Autodesk Inventor part; units mm, degrees
(part 9 of 15)
  arc A3906 (-13.7068, -39.825) -> (-13.6432, -39.825) centre (-13.675, -39.825) ccw
  arc A3907 (-13.6432, -38.375) -> (-13.7068, -38.375) centre (-13.675, -38.375) ccw
  arc A3908 (-15.8, -38.8) -> (-15.8, -38.6) centre (-15.8, -38.7) ccw
  arc A3909 (-15.8, -38.6) -> (-15.8, -38.8) centre (-15.8, -38.7) ccw
  line L1786 (-16.125, -36.575) -> (-13.675, -36.575)
  arc A3910 (-13.675, -36.6067) -> (-13.675, -36.5432) centre (-13.675, -36.575) ccw
  arc A3911 (-16.125, -36.5432) -> (-16.125, -36.6067) centre (-16.125, -36.575) ccw
  line L1787 (-13.675, -38.025) -> (-16.125, -38.025)
  arc A3912 (-16.125, -37.9932) -> (-16.125, -38.0567) centre (-16.125, -38.025) ccw
  arc A3913 (-13.675, -38.0567) -> (-13.675, -37.9932) centre (-13.675, -38.025) ccw
  line L1788 (-16.125, -38.025) -> (-16.125, -36.575)
  arc A3914 (-16.0933, -36.575) -> (-16.1568, -36.575) centre (-16.1251, -36.575) ccw
  arc A3915 (-16.1568, -38.025) -> (-16.0933, -38.025) centre (-16.1251, -38.025) ccw
  line L1789 (-13.675, -36.575) -> (-13.675, -38.025)
  arc A3916 (-13.7068, -38.025) -> (-13.6432, -38.025) centre (-13.675, -38.025) ccw
  arc A3917 (-13.6432, -36.575) -> (-13.7068, -36.575) centre (-13.675, -36.575) ccw
  arc A3918 (-15.8, -37) -> (-15.8, -36.8) centre (-15.8, -36.9) ccw
  arc A3919 (-15.8, -36.8) -> (-15.8, -37) centre (-15.8, -36.9) ccw
  line L1790 (-7.125, -38.375) -> (-4.675, -38.375)
  arc A3920 (-4.675, -38.4067) -> (-4.675, -38.3432) centre (-4.675, -38.375) ccw
  arc A3921 (-7.125, -38.3432) -> (-7.125, -38.4067) centre (-7.125, -38.375) ccw
  line L1791 (-4.675, -39.825) -> (-7.125, -39.825)
  arc A3922 (-7.125, -39.7932) -> (-7.125, -39.8567) centre (-7.125, -39.825) ccw
  arc A3923 (-4.675, -39.8567) -> (-4.675, -39.7932) centre (-4.675, -39.825) ccw
  line L1792 (-7.125, -39.825) -> (-7.125, -38.375)
  arc A3924 (-7.0933, -38.375) -> (-7.1568, -38.375) centre (-7.1251, -38.375) ccw
  arc A3925 (-7.1568, -39.825) -> (-7.0933, -39.825) centre (-7.1251, -39.825) ccw
  line L1793 (-4.675, -38.375) -> (-4.675, -39.825)
  arc A3926 (-4.7068, -39.825) -> (-4.6432, -39.825) centre (-4.675, -39.825) ccw
  arc A3927 (-4.6432, -38.375) -> (-4.7068, -38.375) centre (-4.675, -38.375) ccw
  arc A3928 (-6.8, -38.8) -> (-6.8, -38.6) centre (-6.8, -38.7) ccw
  arc A3929 (-6.8, -38.6) -> (-6.8, -38.8) centre (-6.8, -38.7) ccw
  line L1794 (-7.125, -36.575) -> (-4.675, -36.575)
  arc A3930 (-4.675, -36.6067) -> (-4.675, -36.5432) centre (-4.675, -36.575) ccw
  arc A3931 (-7.125, -36.5432) -> (-7.125, -36.6067) centre (-7.125, -36.575) ccw
  line L1795 (-4.675, -38.025) -> (-7.125, -38.025)
  arc A3932 (-7.125, -37.9932) -> (-7.125, -38.0567) centre (-7.125, -38.025) ccw
  arc A3933 (-4.675, -38.0567) -> (-4.675, -37.9932) centre (-4.675, -38.025) ccw
  line L1796 (-7.125, -38.025) -> (-7.125, -36.575)
  arc A3934 (-7.0933, -36.575) -> (-7.1568, -36.575) centre (-7.1251, -36.575) ccw
  arc A3935 (-7.1568, -38.025) -> (-7.0933, -38.025) centre (-7.1251, -38.025) ccw
  line L1797 (-4.675, -36.575) -> (-4.675, -38.025)
  arc A3936 (-4.7068, -38.025) -> (-4.6432, -38.025) centre (-4.675, -38.025) ccw
  arc A3937 (-4.6432, -36.575) -> (-4.7068, -36.575) centre (-4.675, -36.575) ccw
  arc A3938 (-6.8, -37) -> (-6.8, -36.8) centre (-6.8, -36.9) ccw
  arc A3939 (-6.8, -36.8) -> (-6.8, -37) centre (-6.8, -36.9) ccw
  line L1798 (15.725, -39.725) -> (13.275, -39.725)
  arc A3940 (13.275, -39.6932) -> (13.275, -39.7568) centre (13.275, -39.725) ccw
  arc A3941 (15.725, -39.7568) -> (15.725, -39.6932) centre (15.725, -39.725) ccw
  line L1799 (13.275, -38.275) -> (15.725, -38.275)
  arc A3942 (15.725, -38.3067) -> (15.725, -38.2432) centre (15.725, -38.275) ccw
  arc A3943 (13.275, -38.2432) -> (13.275, -38.3067) centre (13.275, -38.275) ccw
  line L1800 (15.725, -38.275) -> (15.725, -39.725)
  arc A3944 (15.6933, -39.725) -> (15.7568, -39.725) centre (15.725, -39.725) ccw
  arc A3945 (15.7568, -38.275) -> (15.6933, -38.275) centre (15.725, -38.275) ccw
  line L1801 (13.275, -39.725) -> (13.275, -38.275)
  arc A3946 (13.3068, -38.275) -> (13.2433, -38.275) centre (13.275, -38.275) ccw
  arc A3947 (13.2433, -39.725) -> (13.3068, -39.725) centre (13.275, -39.725) ccw
  arc A3948 (15.4, -39.5) -> (15.4, -39.3) centre (15.4, -39.4) ccw
  arc A3949 (15.4, -39.3) -> (15.4, -39.5) centre (15.4, -39.4) ccw
  line L1802 (15.725, -41.625) -> (13.275, -41.625)
  arc A3950 (13.275, -41.5932) -> (13.275, -41.6567) centre (13.275, -41.625) ccw
  arc A3951 (15.725, -41.6567) -> (15.725, -41.5932) centre (15.725, -41.625) ccw
  line L1803 (13.275, -40.175) -> (15.725, -40.175)
  arc A3952 (15.725, -40.2068) -> (15.725, -40.1433) centre (15.725, -40.1751) ccw
  arc A3953 (13.275, -40.1433) -> (13.275, -40.2068) centre (13.275, -40.1751) ccw
  line L1804 (15.725, -40.175) -> (15.725, -41.625)
  arc A3954 (15.6933, -41.625) -> (15.7568, -41.625) centre (15.725, -41.625) ccw
  arc A3955 (15.7568, -40.175) -> (15.6933, -40.175) centre (15.725, -40.175) ccw
  line L1805 (13.275, -41.625) -> (13.275, -40.175)
  arc A3956 (13.3068, -40.175) -> (13.2433, -40.175) centre (13.275, -40.175) ccw
  arc A3957 (13.2433, -41.625) -> (13.3068, -41.625) centre (13.275, -41.625) ccw
  arc A3958 (15.4, -41.4) -> (15.4, -41.2) centre (15.4, -41.3) ccw
  arc A3959 (15.4, -41.2) -> (15.4, -41.4) centre (15.4, -41.3) ccw
  line L1806 (-12.722, -87.325) -> (-12.722, -86.44)
  arc A3960 (-12.6839, -86.44) -> (-12.7601, -86.44) centre (-12.722, -86.44) ccw
  arc A3961 (-12.7601, -87.325) -> (-12.6839, -87.325) centre (-12.722, -87.325) ccw
  line L1807 (-9.878, -86.44) -> (-9.878, -87.325)
  arc A3962 (-9.9161, -87.325) -> (-9.8399, -87.325) centre (-9.878, -87.325) ccw
  arc A3963 (-9.8399, -86.44) -> (-9.9161, -86.44) centre (-9.878, -86.44) ccw
  line L1808 (-12.722, -86.44) -> (-12.018, -86.44)
  arc A3964 (-12.018, -86.4781) -> (-12.018, -86.4019) centre (-12.018, -86.44) ccw
  arc A3965 (-12.722, -86.4019) -> (-12.722, -86.4781) centre (-12.722, -86.44) ccw
  line L1809 (-10.948, -87.76) -> (-11.652, -87.76)
  arc A3966 (-11.652, -87.7219) -> (-11.652, -87.7981) centre (-11.652, -87.76) ccw
  arc A3967 (-10.948, -87.7981) -> (-10.948, -87.7219) centre (-10.948, -87.76) ccw
  line L1810 (-10.582, -86.44) -> (-9.878, -86.44)
  arc A3968 (-9.878, -86.4781) -> (-9.878, -86.4019) centre (-9.878, -86.44) ccw
  arc A3969 (-10.582, -86.4019) -> (-10.582, -86.4781) centre (-10.582, -86.44) ccw
  line L1811 (10.15, -94.475) -> (10.15, -95.125)
  arc A3970 (10.1119, -95.125) -> (10.1881, -95.125) centre (10.15, -95.125) ccw
  arc A3971 (10.1881, -94.475) -> (10.1119, -94.475) centre (10.15, -94.475) ccw
  line L1812 (8.45, -95.125) -> (8.45, -94.475)
  arc A3972 (8.4881, -94.475) -> (8.4119, -94.475) centre (8.45, -94.475) ccw
  arc A3973 (8.4119, -95.125) -> (8.4881, -95.125) centre (8.45, -95.125) ccw
  line L1813 (10.15, -95.125) -> (9.718, -95.125)
  arc A3974 (9.718, -95.0869) -> (9.718, -95.1631) centre (9.718, -95.125) ccw
  arc A3975 (10.15, -95.1631) -> (10.15, -95.0869) centre (10.15, -95.125) ccw
  line L1814 (9.248, -94.275) -> (9.352, -94.275)
  arc A3976 (9.352, -94.3131) -> (9.352, -94.2369) centre (9.352, -94.275) ccw
  arc A3977 (9.248, -94.2369) -> (9.248, -94.3131) centre (9.248, -94.275) ccw
  line L1815 (8.882, -95.125) -> (8.45, -95.125)
  arc A3978 (8.45, -95.0869) -> (8.45, -95.1631) centre (8.45, -95.125) ccw
  arc A3979 (8.882, -95.1631) -> (8.882, -95.0869) centre (8.882, -95.125) ccw
  line L1816 (-8.95, -105.475) -> (-8.95, -106.125)
  arc A3980 (-8.9881, -106.125) -> (-8.9119, -106.125) centre (-8.95, -106.125) ccw
  arc A3981 (-8.9119, -105.475) -> (-8.9881, -105.475) centre (-8.95, -105.475) ccw
  line L1817 (-10.65, -106.125) -> (-10.65, -105.475)
  arc A3982 (-10.6119, -105.475) -> (-10.6881, -105.475) centre (-10.65, -105.475) ccw
  arc A3983 (-10.6881, -106.125) -> (-10.6119, -106.125) centre (-10.65, -106.125) ccw
  line L1818 (-8.95, -106.125) -> (-9.382, -106.125)
  arc A3984 (-9.382, -106.0869) -> (-9.382, -106.1631) centre (-9.382, -106.125) ccw
  arc A3985 (-8.95, -106.1631) -> (-8.95, -106.0869) centre (-8.95, -106.125) ccw
  line L1819 (-9.852, -105.275) -> (-9.748, -105.275)
  arc A3986 (-9.748, -105.3131) -> (-9.748, -105.2369) centre (-9.748, -105.275) ccw
  arc A3987 (-9.852, -105.2369) -> (-9.852, -105.3131) centre (-9.852, -105.275) ccw
  line L1820 (-10.218, -106.125) -> (-10.65, -106.125)
  arc A3988 (-10.65, -106.0869) -> (-10.65, -106.1631) centre (-10.65, -106.125) ccw
  arc A3989 (-10.218, -106.1631) -> (-10.218, -106.0869) centre (-10.218, -106.125) ccw
  line L1821 (10.15, -92.575) -> (10.15, -93.225)
  arc A3990 (10.1119, -93.225) -> (10.1881, -93.225) centre (10.15, -93.225) ccw
  arc A3991 (10.1881, -92.575) -> (10.1119, -92.575) centre (10.15, -92.575) ccw
  line L1822 (8.45, -93.225) -> (8.45, -92.575)
  arc A3992 (8.4881, -92.575) -> (8.4119, -92.575) centre (8.45, -92.575) ccw
  arc A3993 (8.4119, -93.225) -> (8.4881, -93.225) centre (8.45, -93.225) ccw
  line L1823 (10.15, -93.225) -> (9.718, -93.225)
  arc A3994 (9.718, -93.1869) -> (9.718, -93.2631) centre (9.718, -93.225) ccw
  arc A3995 (10.15, -93.2631) -> (10.15, -93.1869) centre (10.15, -93.225) ccw
  line L1824 (9.248, -92.375) -> (9.352, -92.375)
  arc A3996 (9.352, -92.4131) -> (9.352, -92.3369) centre (9.352, -92.375) ccw
  arc A3997 (9.248, -92.3369) -> (9.248, -92.4131) centre (9.248, -92.375) ccw
  line L1825 (8.882, -93.225) -> (8.45, -93.225)
  arc A3998 (8.45, -93.1869) -> (8.45, -93.2631) centre (8.45, -93.225) ccw
  arc A3999 (8.882, -93.2631) -> (8.882, -93.1869) centre (8.882, -93.225) ccw
  line L1826 (-8.95, -107.475) -> (-8.95, -108.125)
  arc A4000 (-8.9881, -108.125) -> (-8.9119, -108.125) centre (-8.95, -108.125) ccw
  arc A4001 (-8.9119, -107.475) -> (-8.9881, -107.475) centre (-8.95, -107.475) ccw
  line L1827 (-10.65, -108.125) -> (-10.65, -107.475)
  arc A4002 (-10.6119, -107.475) -> (-10.6881, -107.475) centre (-10.65, -107.475) ccw
  arc A4003 (-10.6881, -108.125) -> (-10.6119, -108.125) centre (-10.65, -108.125) ccw
  line L1828 (-8.95, -108.125) -> (-9.382, -108.125)
  arc A4004 (-9.382, -108.0869) -> (-9.382, -108.1631) centre (-9.382, -108.125) ccw
  arc A4005 (-8.95, -108.1631) -> (-8.95, -108.0869) centre (-8.95, -108.125) ccw
  line L1829 (-9.852, -107.275) -> (-9.748, -107.275)
  arc A4006 (-9.748, -107.3131) -> (-9.748, -107.2369) centre (-9.748, -107.275) ccw
  arc A4007 (-9.852, -107.2369) -> (-9.852, -107.3131) centre (-9.852, -107.275) ccw
  line L1830 (-10.218, -108.125) -> (-10.65, -108.125)
  arc A4008 (-10.65, -108.0869) -> (-10.65, -108.1631) centre (-10.65, -108.125) ccw
  arc A4009 (-10.218, -108.1631) -> (-10.218, -108.0869) centre (-10.218, -108.125) ccw
  line L1831 (19.75, -91.825) -> (19.75, -91.175)
  arc A4010 (19.7881, -91.175) -> (19.7119, -91.175) centre (19.75, -91.175) ccw
  arc A4011 (19.7119, -91.825) -> (19.7881, -91.825) centre (19.75, -91.825) ccw
  line L1832 (21.45, -91.175) -> (21.45, -91.825)
  arc A4012 (21.4119, -91.825) -> (21.4881, -91.825) centre (21.45, -91.825) ccw
  arc A4013 (21.4881, -91.175) -> (21.4119, -91.175) centre (21.45, -91.175) ccw
  line L1833 (19.75, -91.175) -> (20.182, -91.175)
  arc A4014 (20.182, -91.2131) -> (20.182, -91.1369) centre (20.182, -91.175) ccw
  arc A4015 (19.75, -91.1369) -> (19.75, -91.2131) centre (19.75, -91.175) ccw
  line L1834 (20.652, -92.025) -> (20.548, -92.025)
  arc A4016 (20.548, -91.9869) -> (20.548, -92.0631) centre (20.548, -92.025) ccw
  arc A4017 (20.652, -92.0631) -> (20.652, -91.9869) centre (20.652, -92.025) ccw
  line L1835 (21.018, -91.175) -> (21.45, -91.175)
  arc A4018 (21.45, -91.2131) -> (21.45, -91.1369) centre (21.45, -91.175) ccw
  arc A4019 (21.018, -91.1369) -> (21.018, -91.2131) centre (21.018, -91.175) ccw
  line L1836 (19.75, -94.925) -> (19.75, -94.275)
  arc A4020 (19.7881, -94.275) -> (19.7119, -94.275) centre (19.75, -94.275) ccw
  arc A4021 (19.7119, -94.925) -> (19.7881, -94.925) centre (19.75, -94.925) ccw
  line L1837 (21.45, -94.275) -> (21.45, -94.925)
  arc A4022 (21.4119, -94.925) -> (21.4881, -94.925) centre (21.45, -94.925) ccw
  arc A4023 (21.4881, -94.275) -> (21.4119, -94.275) centre (21.45, -94.275) ccw
  line L1838 (19.75, -94.275) -> (20.182, -94.275)
  arc A4024 (20.182, -94.3131) -> (20.182, -94.2369) centre (20.182, -94.275) ccw
  arc A4025 (19.75, -94.2369) -> (19.75, -94.3131) centre (19.75, -94.275) ccw
  line L1839 (20.652, -95.125) -> (20.548, -95.125)
  arc A4026 (20.548, -95.0869) -> (20.548, -95.1631) centre (20.548, -95.125) ccw
  arc A4027 (20.652, -95.1631) -> (20.652, -95.0869) centre (20.652, -95.125) ccw
  line L1840 (21.018, -94.275) -> (21.45, -94.275)
  arc A4028 (21.45, -94.3131) -> (21.45, -94.2369) centre (21.45, -94.275) ccw
  arc A4029 (21.018, -94.2369) -> (21.018, -94.3131) centre (21.018, -94.275) ccw
  line L1841 (21.75, -94.925) -> (21.75, -94.275)
  arc A4030 (21.7881, -94.275) -> (21.7119, -94.275) centre (21.75, -94.275) ccw
  arc A4031 (21.7119, -94.925) -> (21.7881, -94.925) centre (21.75, -94.925) ccw
  line L1842 (23.45, -94.275) -> (23.45, -94.925)
  arc A4032 (23.4119, -94.925) -> (23.4881, -94.925) centre (23.45, -94.925) ccw
  arc A4033 (23.4881, -94.275) -> (23.4119, -94.275) centre (23.45, -94.275) ccw
  line L1843 (21.75, -94.275) -> (22.182, -94.275)
  arc A4034 (22.182, -94.3131) -> (22.182, -94.2369) centre (22.182, -94.275) ccw
  arc A4035 (21.75, -94.2369) -> (21.75, -94.3131) centre (21.75, -94.275) ccw
  line L1844 (22.652, -95.125) -> (22.548, -95.125)
  arc A4036 (22.548, -95.0869) -> (22.548, -95.1631) centre (22.548, -95.125) ccw
  arc A4037 (22.652, -95.1631) -> (22.652, -95.0869) centre (22.652, -95.125) ccw
  line L1845 (23.018, -94.275) -> (23.45, -94.275)
  arc A4038 (23.45, -94.3131) -> (23.45, -94.2369) centre (23.45, -94.275) ccw
  arc A4039 (23.018, -94.2369) -> (23.018, -94.3131) centre (23.018, -94.275) ccw
  line L1846 (21.75, -91.825) -> (21.75, -91.175)
  arc A4040 (21.7881, -91.175) -> (21.7119, -91.175) centre (21.75, -91.175) ccw
  arc A4041 (21.7119, -91.825) -> (21.7881, -91.825) centre (21.75, -91.825) ccw
  line L1847 (23.45, -91.175) -> (23.45, -91.825)
  arc A4042 (23.4119, -91.825) -> (23.4881, -91.825) centre (23.45, -91.825) ccw
  arc A4043 (23.4881, -91.175) -> (23.4119, -91.175) centre (23.45, -91.175) ccw
  line L1848 (21.75, -91.175) -> (22.182, -91.175)
  arc A4044 (22.182, -91.2131) -> (22.182, -91.1369) centre (22.182, -91.175) ccw
  arc A4045 (21.75, -91.1369) -> (21.75, -91.2131) centre (21.75, -91.175) ccw
  line L1849 (22.652, -92.025) -> (22.548, -92.025)
  arc A4046 (22.548, -91.9869) -> (22.548, -92.0631) centre (22.548, -92.025) ccw
  arc A4047 (22.652, -92.0631) -> (22.652, -91.9869) centre (22.652, -92.025) ccw
  line L1850 (23.018, -91.175) -> (23.45, -91.175)
  arc A4048 (23.45, -91.2131) -> (23.45, -91.1369) centre (23.45, -91.175) ccw
  arc A4049 (23.018, -91.1369) -> (23.018, -91.2131) centre (23.018, -91.175) ccw
  line L1851 (-55.4108, -61.543) -> (-60.3892, -61.543)
  arc A4050 (-60.3892, -61.4922) -> (-60.3892, -61.5938) centre (-60.3892, -61.543) ccw
  arc A4051 (-55.4108, -61.5938) -> (-55.4108, -61.4922) centre (-55.4108, -61.543) ccw
  line L1852 (-60.3892, -61.543) -> (-60.3892, -59.257)
  arc A4052 (-60.3384, -59.257) -> (-60.44, -59.257) centre (-60.3892, -59.257) ccw
  arc A4053 (-60.44, -61.543) -> (-60.3384, -61.543) centre (-60.3892, -61.543) ccw
  line L1853 (-60.3892, -59.257) -> (-55.4108, -59.257)
  arc A4054 (-55.4108, -59.3078) -> (-55.4108, -59.2062) centre (-55.4108, -59.257) ccw
  arc A4055 (-60.3892, -59.2062) -> (-60.3892, -59.3078) centre (-60.3892, -59.257) ccw
  line L1854 (-55.4108, -59.257) -> (-55.4108, -61.543)
  arc A4056 (-55.4616, -61.543) -> (-55.36, -61.543) centre (-55.4108, -61.543) ccw
  arc A4057 (-55.36, -59.257) -> (-55.4616, -59.257) centre (-55.4108, -59.257) ccw
  line L1855 (-10.2542, 51.989) -> (-6.5458, 51.989)
  arc A4058 (-6.5458, 51.9382) -> (-6.5458, 52.0398) centre (-6.5458, 51.989) ccw
  arc A4059 (-10.2542, 52.0398) -> (-10.2542, 51.9382) centre (-10.2542, 51.989) ccw
  line L1856 (-6.5458, 51.989) -> (-6.5458, 50.211)
  arc A4060 (-6.5966, 50.211) -> (-6.495, 50.211) centre (-6.5458, 50.211) ccw
  arc A4061 (-6.495, 51.989) -> (-6.5966, 51.989) centre (-6.5458, 51.989) ccw
  line L1857 (-6.5458, 50.211) -> (-10.2542, 50.211)
  arc A4062 (-10.2542, 50.2618) -> (-10.2542, 50.1602) centre (-10.2542, 50.211) ccw
  arc A4063 (-6.5458, 50.1602) -> (-6.5458, 50.2618) centre (-6.5458, 50.211) ccw
  line L1858 (-10.2542, 50.211) -> (-10.2542, 51.989)
  arc A4064 (-10.2034, 51.989) -> (-10.305, 51.989) centre (-10.2542, 51.989) ccw
  arc A4065 (-10.305, 50.211) -> (-10.2034, 50.211) centre (-10.2542, 50.211) ccw
  line L1859 (-7.692, -83.684) -> (-7.692, -85.716)
  arc A4066 (-7.7428, -85.716) -> (-7.6412, -85.716) centre (-7.692, -85.716) ccw
  arc A4067 (-7.6412, -83.684) -> (-7.7428, -83.684) centre (-7.692, -83.684) ccw
  line L1860 (-7.692, -85.716) -> (-8.708, -85.716)
  arc A4068 (-8.708, -85.6652) -> (-8.708, -85.7668) centre (-8.708, -85.716) ccw
  arc A4069 (-7.692, -85.7668) -> (-7.692, -85.6652) centre (-7.692, -85.716) ccw
  line L1861 (-8.708, -85.716) -> (-8.708, -83.684)
  arc A4070 (-8.6572, -83.684) -> (-8.7588, -83.684) centre (-8.708, -83.684) ccw
  arc A4071 (-8.7588, -85.716) -> (-8.6572, -85.716) centre (-8.708, -85.716) ccw
  line L1862 (-8.708, -83.684) -> (-7.692, -83.684)
  arc A4072 (-7.692, -83.7348) -> (-7.692, -83.6332) centre (-7.692, -83.684) ccw
  arc A4073 (-8.708, -83.6332) -> (-8.708, -83.7348) centre (-8.708, -83.684) ccw
  line L1863 (-5.5458, -87.889) -> (-9.2542, -87.889)
  arc A4074 (-9.2542, -87.8382) -> (-9.2542, -87.9398) centre (-9.2542, -87.889) ccw
  arc A4075 (-5.5458, -87.9398) -> (-5.5458, -87.8382) centre (-5.5458, -87.889) ccw
  line L1864 (-9.2542, -87.889) -> (-9.2542, -86.111)
  arc A4076 (-9.2034, -86.111) -> (-9.305, -86.111) centre (-9.2542, -86.111) ccw
  arc A4077 (-9.305, -87.889) -> (-9.2034, -87.889) centre (-9.2542, -87.889) ccw
  line L1865 (-9.2542, -86.111) -> (-5.5458, -86.111)
  arc A4078 (-5.5458, -86.1618) -> (-5.5458, -86.0602) centre (-5.5458, -86.111) ccw
  arc A4079 (-9.2542, -86.0602) -> (-9.2542, -86.1618) centre (-9.2542, -86.111) ccw
  line L1866 (-5.5458, -86.111) -> (-5.5458, -87.889)
  arc A4080 (-5.5966, -87.889) -> (-5.495, -87.889) centre (-5.5458, -87.889) ccw
  arc A4081 (-5.495, -86.111) -> (-5.5966, -86.111) centre (-5.5458, -86.111) ccw
  line L1867 (-13.392, -87.984) -> (-13.392, -90.016)
  arc A4082 (-13.4428, -90.016) -> (-13.3412, -90.016) centre (-13.392, -90.016) ccw
  arc A4083 (-13.3412, -87.984) -> (-13.4428, -87.984) centre (-13.392, -87.984) ccw
  line L1868 (-13.392, -90.016) -> (-14.408, -90.016)
  arc A4084 (-14.408, -89.9652) -> (-14.408, -90.0668) centre (-14.408, -90.016) ccw
  arc A4085 (-13.392, -90.0668) -> (-13.392, -89.9652) centre (-13.392, -90.016) ccw
  line L1869 (-14.408, -90.016) -> (-14.408, -87.984)
  arc A4086 (-14.3572, -87.984) -> (-14.4588, -87.984) centre (-14.408, -87.984) ccw
  arc A4087 (-14.4588, -90.016) -> (-14.3572, -90.016) centre (-14.408, -90.016) ccw
  line L1870 (-14.408, -87.984) -> (-13.392, -87.984)
  arc A4088 (-13.392, -88.0348) -> (-13.392, -87.9332) centre (-13.392, -87.984) ccw
  arc A4089 (-14.408, -87.9332) -> (-14.408, -88.0348) centre (-14.408, -87.984) ccw
  line L1871 (-9.3458, -90.889) -> (-13.0542, -90.889)
  arc A4090 (-13.0542, -90.8382) -> (-13.0542, -90.9398) centre (-13.0542, -90.889) ccw
  arc A4091 (-9.3458, -90.9398) -> (-9.3458, -90.8382) centre (-9.3458, -90.889) ccw
  line L1872 (-13.0542, -90.889) -> (-13.0542, -89.111)
  arc A4092 (-13.0034, -89.111) -> (-13.105, -89.111) centre (-13.0542, -89.111) ccw
  arc A4093 (-13.105, -90.889) -> (-13.0034, -90.889) centre (-13.0542, -90.889) ccw
  line L1873 (-13.0542, -89.111) -> (-9.3458, -89.111)
  arc A4094 (-9.3458, -89.1618) -> (-9.3458, -89.0602) centre (-9.3458, -89.111) ccw
  arc A4095 (-13.0542, -89.0602) -> (-13.0542, -89.1618) centre (-13.0542, -89.111) ccw
  line L1874 (-9.3458, -89.111) -> (-9.3458, -90.889)
  arc A4096 (-9.3966, -90.889) -> (-9.295, -90.889) centre (-9.3458, -90.889) ccw
  arc A4097 (-9.295, -89.111) -> (-9.3966, -89.111) centre (-9.3458, -89.111) ccw
  line L1875 (-13.303, -97.035) -> (-16.097, -97.035)
  arc A4098 (-16.097, -96.9842) -> (-16.097, -97.0858) centre (-16.097, -97.035) ccw
  arc A4099 (-13.303, -97.0858) -> (-13.303, -96.9842) centre (-13.303, -97.035) ccw
  line L1876 (-16.097, -97.035) -> (-16.097, -95.765)
  arc A4100 (-16.0462, -95.765) -> (-16.1478, -95.765) centre (-16.097, -95.765) ccw
  arc A4101 (-16.1478, -97.035) -> (-16.0462, -97.035) centre (-16.097, -97.035) ccw
  line L1877 (-16.097, -95.765) -> (-13.303, -95.765)
  arc A4102 (-13.303, -95.8158) -> (-13.303, -95.7142) centre (-13.303, -95.765) ccw
  arc A4103 (-16.097, -95.7142) -> (-16.097, -95.8158) centre (-16.097, -95.765) ccw
  line L1878 (-13.303, -95.765) -> (-13.303, -97.035)
  arc A4104 (-13.3538, -97.035) -> (-13.2522, -97.035) centre (-13.303, -97.035) ccw
  arc A4105 (-13.2522, -95.765) -> (-13.3538, -95.765) centre (-13.303, -95.765) ccw
  line L1879 (-18.316, -98.092) -> (-16.284, -98.092)
  arc A4106 (-16.284, -98.1428) -> (-16.284, -98.0412) centre (-16.284, -98.092) ccw
  arc A4107 (-18.316, -98.0412) -> (-18.316, -98.1428) centre (-18.316, -98.092) ccw
  line L1880 (-16.284, -98.092) -> (-16.284, -99.108)
  arc A4108 (-16.3348, -99.108) -> (-16.2332, -99.108) centre (-16.284, -99.108) ccw
  arc A4109 (-16.2332, -98.092) -> (-16.3348, -98.092) centre (-16.284, -98.092) ccw
  line L1881 (-16.284, -99.108) -> (-18.316, -99.108)
  arc A4110 (-18.316, -99.0572) -> (-18.316, -99.1588) centre (-18.316, -99.108) ccw
  arc A4111 (-16.284, -99.1588) -> (-16.284, -99.0572) centre (-16.284, -99.108) ccw
  line L1882 (-18.316, -99.108) -> (-18.316, -98.092)
  arc A4112 (-18.2652, -98.092) -> (-18.3668, -98.092) centre (-18.316, -98.092) ccw
  arc A4113 (-18.3668, -99.108) -> (-18.2652, -99.108) centre (-18.316, -99.108) ccw
  line L1883 (-17.284, -103.108) -> (-19.316, -103.108)
  arc A4114 (-19.316, -103.0572) -> (-19.316, -103.1588) centre (-19.316, -103.108) ccw
  arc A4115 (-17.284, -103.1588) -> (-17.284, -103.0572) centre (-17.284, -103.108) ccw
  line L1884 (-19.316, -103.108) -> (-19.316, -102.092)
  arc A4116 (-19.2652, -102.092) -> (-19.3668, -102.092) centre (-19.316, -102.092) ccw
  arc A4117 (-19.3668, -103.108) -> (-19.2652, -103.108) centre (-19.316, -103.108) ccw
  line L1885 (-19.316, -102.092) -> (-17.284, -102.092)
  arc A4118 (-17.284, -102.1428) -> (-17.284, -102.0412) centre (-17.284, -102.092) ccw
  arc A4119 (-19.316, -102.0412) -> (-19.316, -102.1428) centre (-19.316, -102.092) ccw
  line L1886 (-17.284, -102.092) -> (-17.284, -103.108)
  arc A4120 (-17.3348, -103.108) -> (-17.2332, -103.108) centre (-17.284, -103.108) ccw
  arc A4121 (-17.2332, -102.092) -> (-17.3348, -102.092) centre (-17.284, -102.092) ccw
  line L1887 (-17.308, -105.116) -> (-17.308, -103.084)
  arc A4122 (-17.2572, -103.084) -> (-17.3588, -103.084) centre (-17.308, -103.084) ccw
  arc A4123 (-17.3588, -105.116) -> (-17.2572, -105.116) centre (-17.308, -105.116) ccw
  line L1888 (-17.308, -103.084) -> (-16.292, -103.084)
  arc A4124 (-16.292, -103.1348) -> (-16.292, -103.0332) centre (-16.292, -103.084) ccw
  arc A4125 (-17.308, -103.0332) -> (-17.308, -103.1348) centre (-17.308, -103.084) ccw
  line L1889 (-16.292, -103.084) -> (-16.292, -105.116)
  arc A4126 (-16.3428, -105.116) -> (-16.2412, -105.116) centre (-16.292, -105.116) ccw
  arc A4127 (-16.2412, -103.084) -> (-16.3428, -103.084) centre (-16.292, -103.084) ccw
  line L1890 (-16.292, -105.116) -> (-17.308, -105.116)
  arc A4128 (-17.308, -105.0652) -> (-17.308, -105.1668) centre (-17.308, -105.116) ccw
  arc A4129 (-16.292, -105.1668) -> (-16.292, -105.0652) centre (-16.292, -105.116) ccw
  line L1891 (-19.308, -105.116) -> (-19.308, -103.084)
  arc A4130 (-19.2572, -103.084) -> (-19.3588, -103.084) centre (-19.308, -103.084) ccw
  arc A4131 (-19.3588, -105.116) -> (-19.2572, -105.116) centre (-19.308, -105.116) ccw
  line L1892 (-19.308, -103.084) -> (-18.292, -103.084)
  arc A4132 (-18.292, -103.1348) -> (-18.292, -103.0332) centre (-18.292, -103.084) ccw
  arc A4133 (-19.308, -103.0332) -> (-19.308, -103.1348) centre (-19.308, -103.084) ccw
  line L1893 (-18.292, -103.084) -> (-18.292, -105.116)
  arc A4134 (-18.3428, -105.116) -> (-18.2412, -105.116) centre (-18.292, -105.116) ccw
  arc A4135 (-18.2412, -103.084) -> (-18.3428, -103.084) centre (-18.292, -103.084) ccw
  line L1894 (-18.292, -105.116) -> (-19.308, -105.116)
  arc A4136 (-19.308, -105.0652) -> (-19.308, -105.1668) centre (-19.308, -105.116) ccw
  arc A4137 (-18.292, -105.1668) -> (-18.292, -105.0652) centre (-18.292, -105.116) ccw
  line L1895 (-19.308, -102.116) -> (-19.308, -100.084)
  arc A4138 (-19.2572, -100.084) -> (-19.3588, -100.084) centre (-19.308, -100.084) ccw
  arc A4139 (-19.3588, -102.116) -> (-19.2572, -102.116) centre (-19.308, -102.116) ccw
  line L1896 (-19.308, -100.084) -> (-18.292, -100.084)
  arc A4140 (-18.292, -100.1348) -> (-18.292, -100.0332) centre (-18.292, -100.084) ccw
  arc A4141 (-19.308, -100.0332) -> (-19.308, -100.1348) centre (-19.308, -100.084) ccw
  line L1897 (-18.292, -100.084) -> (-18.292, -102.116)
  arc A4142 (-18.3428, -102.116) -> (-18.2412, -102.116) centre (-18.292, -102.116) ccw
  arc A4143 (-18.2412, -100.084) -> (-18.3428, -100.084) centre (-18.292, -100.084) ccw
  line L1898 (-18.292, -102.116) -> (-19.308, -102.116)
  arc A4144 (-19.308, -102.0652) -> (-19.308, -102.1668) centre (-19.308, -102.116) ccw
  arc A4145 (-18.292, -102.1668) -> (-18.292, -102.0652) centre (-18.292, -102.116) ccw
  line L1899 (-18.308, -98.116) -> (-18.308, -96.084)
  arc A4146 (-18.2572, -96.084) -> (-18.3588, -96.084) centre (-18.308, -96.084) ccw
  arc A4147 (-18.3588, -98.116) -> (-18.2572, -98.116) centre (-18.308, -98.116) ccw
  line L1900 (-18.308, -96.084) -> (-17.292, -96.084)
  arc A4148 (-17.292, -96.1348) -> (-17.292, -96.0332) centre (-17.292, -96.084) ccw
  arc A4149 (-18.308, -96.0332) -> (-18.308, -96.1348) centre (-18.308, -96.084) ccw
  line L1901 (-17.292, -96.084) -> (-17.292, -98.116)
  arc A4150 (-17.3428, -98.116) -> (-17.2412, -98.116) centre (-17.292, -98.116) ccw
  arc A4151 (-17.2412, -96.084) -> (-17.3428, -96.084) centre (-17.292, -96.084) ccw
  line L1902 (-17.292, -98.116) -> (-18.308, -98.116)
  arc A4152 (-18.308, -98.0652) -> (-18.308, -98.1668) centre (-18.308, -98.116) ccw
  arc A4153 (-17.292, -98.1668) -> (-17.292, -98.0652) centre (-17.292, -98.116) ccw
  line L1903 (-16.208, -105.116) -> (-16.208, -103.084)
  arc A4154 (-16.1572, -103.084) -> (-16.2588, -103.084) centre (-16.208, -103.084) ccw
  arc A4155 (-16.2588, -105.116) -> (-16.1572, -105.116) centre (-16.208, -105.116) ccw
  line L1904 (-16.208, -103.084) -> (-15.192, -103.084)
  arc A4156 (-15.192, -103.1348) -> (-15.192, -103.0332) centre (-15.192, -103.084) ccw
  arc A4157 (-16.208, -103.0332) -> (-16.208, -103.1348) centre (-16.208, -103.084) ccw
  line L1905 (-15.192, -103.084) -> (-15.192, -105.116)
  arc A4158 (-15.2428, -105.116) -> (-15.1412, -105.116) centre (-15.192, -105.116) ccw
  arc A4159 (-15.1412, -103.084) -> (-15.2428, -103.084) centre (-15.192, -103.084) ccw
  line L1906 (-15.192, -105.116) -> (-16.208, -105.116)
  arc A4160 (-16.208, -105.0652) -> (-16.208, -105.1668) centre (-16.208, -105.116) ccw
  arc A4161 (-15.192, -105.1668) -> (-15.192, -105.0652) centre (-15.192, -105.116) ccw
  line L1907 (-8.365, -97.203) -> (-8.365, -99.997)
  arc A4162 (-8.4158, -99.997) -> (-8.3142, -99.997) centre (-8.365, -99.997) ccw
  arc A4163 (-8.3142, -97.203) -> (-8.4158, -97.203) centre (-8.365, -97.203) ccw
  line L1908 (-8.365, -99.997) -> (-9.635, -99.997)
  arc A4164 (-9.635, -99.9462) -> (-9.635, -100.0478) centre (-9.635, -99.997) ccw
  arc A4165 (-8.365, -100.0478) -> (-8.365, -99.9462) centre (-8.365, -99.997) ccw
  line L1909 (-9.635, -99.997) -> (-9.635, -97.203)
  arc A4166 (-9.5842, -97.203) -> (-9.6858, -97.203) centre (-9.635, -97.203) ccw
  arc A4167 (-9.6858, -99.997) -> (-9.5842, -99.997) centre (-9.635, -99.997) ccw
  line L1910 (-9.635, -97.203) -> (-8.365, -97.203)
  arc A4168 (-8.365, -97.2538) -> (-8.365, -97.1522) centre (-8.365, -97.203) ccw
  arc A4169 (-9.635, -97.1522) -> (-9.635, -97.2538) centre (-9.635, -97.203) ccw
  line L1911 (-10.2542, 50.189) -> (-6.5458, 50.189)
  arc A4170 (-6.5458, 50.1382) -> (-6.5458, 50.2398) centre (-6.5458, 50.189) ccw
  arc A4171 (-10.2542, 50.2398) -> (-10.2542, 50.1382) centre (-10.2542, 50.189) ccw
  line L1912 (-6.5458, 50.189) -> (-6.5458, 48.411)
  arc A4172 (-6.5966, 48.411) -> (-6.495, 48.411) centre (-6.5458, 48.411) ccw
  arc A4173 (-6.495, 50.189) -> (-6.5966, 50.189) centre (-6.5458, 50.189) ccw
  line L1913 (-6.5458, 48.411) -> (-10.2542, 48.411)
  arc A4174 (-10.2542, 48.4618) -> (-10.2542, 48.3602) centre (-10.2542, 48.411) ccw
  arc A4175 (-6.5458, 48.3602) -> (-6.5458, 48.4618) centre (-6.5458, 48.411) ccw
  line L1914 (-10.2542, 48.411) -> (-10.2542, 50.189)
  arc A4176 (-10.2034, 50.189) -> (-10.305, 50.189) centre (-10.2542, 50.189) ccw
  arc A4177 (-10.305, 48.411) -> (-10.2034, 48.411) centre (-10.2542, 48.411) ccw
  line L1915 (-13.792, -107.384) -> (-13.792, -109.416)
  arc A4178 (-13.8428, -109.416) -> (-13.7412, -109.416) centre (-13.792, -109.416) ccw
  arc A4179 (-13.7412, -107.384) -> (-13.8428, -107.384) centre (-13.792, -107.384) ccw
  line L1916 (-13.792, -109.416) -> (-14.808, -109.416)
  arc A4180 (-14.808, -109.3652) -> (-14.808, -109.4668) centre (-14.808, -109.416) ccw
  arc A4181 (-13.792, -109.4668) -> (-13.792, -109.3652) centre (-13.792, -109.416) ccw
  line L1917 (-14.808, -109.416) -> (-14.808, -107.384)
  arc A4182 (-14.7572, -107.384) -> (-14.8588, -107.384) centre (-14.808, -107.384) ccw
  arc A4183 (-14.8588, -109.416) -> (-14.7572, -109.416) centre (-14.808, -109.416) ccw
  line L1918 (-14.808, -107.384) -> (-13.792, -107.384)
  arc A4184 (-13.792, -107.4348) -> (-13.792, -107.3332) centre (-13.792, -107.384) ccw
  arc A4185 (-14.808, -107.3332) -> (-14.808, -107.4348) centre (-14.808, -107.384) ccw
  line L1919 (-15.816, -106.392) -> (-13.784, -106.392)
  arc A4186 (-13.784, -106.4428) -> (-13.784, -106.3412) centre (-13.784, -106.392) ccw
  arc A4187 (-15.816, -106.3412) -> (-15.816, -106.4428) centre (-15.816, -106.392) ccw
  line L1920 (-13.784, -106.392) -> (-13.784, -107.408)
  arc A4188 (-13.8348, -107.408) -> (-13.7332, -107.408) centre (-13.784, -107.408) ccw
  arc A4189 (-13.7332, -106.392) -> (-13.8348, -106.392) centre (-13.784, -106.392) ccw
  line L1921 (-13.784, -107.408) -> (-15.816, -107.408)
  arc A4190 (-15.816, -107.3572) -> (-15.816, -107.4588) centre (-15.816, -107.408) ccw
  arc A4191 (-13.784, -107.4588) -> (-13.784, -107.3572) centre (-13.784, -107.408) ccw
  line L1922 (-15.816, -107.408) -> (-15.816, -106.392)
  arc A4192 (-15.7652, -106.392) -> (-15.8668, -106.392) centre (-15.816, -106.392) ccw
  arc A4193 (-15.8668, -107.408) -> (-15.7652, -107.408) centre (-15.816, -107.408) ccw
  line L1923 (14.216, -85.008) -> (12.184, -85.008)
  arc A4194 (12.184, -84.9572) -> (12.184, -85.0588) centre (12.184, -85.008) ccw
  arc A4195 (14.216, -85.0588) -> (14.216, -84.9572) centre (14.216, -85.008) ccw
  line L1924 (12.184, -85.008) -> (12.184, -83.992)
  arc A4196 (12.2348, -83.992) -> (12.1332, -83.992) centre (12.184, -83.992) ccw
  arc A4197 (12.1332, -85.008) -> (12.2348, -85.008) centre (12.184, -85.008) ccw
  line L1925 (12.184, -83.992) -> (14.216, -83.992)
  arc A4198 (14.216, -84.0428) -> (14.216, -83.9412) centre (14.216, -83.992) ccw
  arc A4199 (12.184, -83.9412) -> (12.184, -84.0428) centre (12.184, -83.992) ccw
  line L1926 (14.216, -83.992) -> (14.216, -85.008)
  arc A4200 (14.1652, -85.008) -> (14.2668, -85.008) centre (14.216, -85.008) ccw
  arc A4201 (14.2668, -83.992) -> (14.1652, -83.992) centre (14.216, -83.992) ccw
  line L1927 (9.584, -82.992) -> (11.616, -82.992)
  arc A4202 (11.616, -83.0428) -> (11.616, -82.9412) centre (11.616, -82.992) ccw
  arc A4203 (9.584, -82.9412) -> (9.584, -83.0428) centre (9.584, -82.992) ccw
  line L1928 (11.616, -82.992) -> (11.616, -84.008)
  arc A4204 (11.5652, -84.008) -> (11.6668, -84.008) centre (11.616, -84.008) ccw
  arc A4205 (11.6668, -82.992) -> (11.5652, -82.992) centre (11.616, -82.992) ccw
  line L1929 (11.616, -84.008) -> (9.584, -84.008)
  arc A4206 (9.584, -83.9572) -> (9.584, -84.0588) centre (9.584, -84.008) ccw
  arc A4207 (11.616, -84.0588) -> (11.616, -83.9572) centre (11.616, -84.008) ccw
  line L1930 (9.584, -84.008) -> (9.584, -82.992)
  arc A4208 (9.6348, -82.992) -> (9.5332, -82.992) centre (9.584, -82.992) ccw
  arc A4209 (9.5332, -84.008) -> (9.6348, -84.008) centre (9.584, -84.008) ccw
  line L1931 (9.584, -81.492) -> (11.616, -81.492)
  arc A4210 (11.616, -81.5428) -> (11.616, -81.4412) centre (11.616, -81.492) ccw
  arc A4211 (9.584, -81.4412) -> (9.584, -81.5428) centre (9.584, -81.492) ccw
  line L1932 (11.616, -81.492) -> (11.616, -82.508)
  arc A4212 (11.5652, -82.508) -> (11.6668, -82.508) centre (11.616, -82.508) ccw
  arc A4213 (11.6668, -81.492) -> (11.5652, -81.492) centre (11.616, -81.492) ccw
  line L1933 (11.616, -82.508) -> (9.584, -82.508)
  arc A4214 (9.584, -82.4572) -> (9.584, -82.5588) centre (9.584, -82.508) ccw
  arc A4215 (11.616, -82.5588) -> (11.616, -82.4572) centre (11.616, -82.508) ccw
  line L1934 (9.584, -82.508) -> (9.584, -81.492)
  arc A4216 (9.6348, -81.492) -> (9.5332, -81.492) centre (9.584, -81.492) ccw
  arc A4217 (9.5332, -82.508) -> (9.6348, -82.508) centre (9.584, -82.508) ccw
  line L1935 (15.292, -88.916) -> (15.292, -86.884)
  arc A4218 (15.3428, -86.884) -> (15.2412, -86.884) centre (15.292, -86.884) ccw
  arc A4219 (15.2412, -88.916) -> (15.3428, -88.916) centre (15.292, -88.916) ccw
  line L1936 (15.292, -86.884) -> (16.308, -86.884)
  arc A4220 (16.308, -86.9348) -> (16.308, -86.8332) centre (16.308, -86.884) ccw
  arc A4221 (15.292, -86.8332) -> (15.292, -86.9348) centre (15.292, -86.884) ccw
  line L1937 (16.308, -86.884) -> (16.308, -88.916)
  arc A4222 (16.2572, -88.916) -> (16.3588, -88.916) centre (16.308, -88.916) ccw
  arc A4223 (16.3588, -86.884) -> (16.2572, -86.884) centre (16.308, -86.884) ccw
  line L1938 (16.308, -88.916) -> (15.292, -88.916)
  arc A4224 (15.292, -88.8652) -> (15.292, -88.9668) centre (15.292, -88.916) ccw
  arc A4225 (16.308, -88.9668) -> (16.308, -88.8652) centre (16.308, -88.916) ccw
  line L1939 (14.092, -88.916) -> (14.092, -86.884)
  arc A4226 (14.1428, -86.884) -> (14.0412, -86.884) centre (14.092, -86.884) ccw
  arc A4227 (14.0412, -88.916) -> (14.1428, -88.916) centre (14.092, -88.916) ccw
  line L1940 (14.092, -86.884) -> (15.108, -86.884)
  arc A4228 (15.108, -86.9348) -> (15.108, -86.8332) centre (15.108, -86.884) ccw
  arc A4229 (14.092, -86.8332) -> (14.092, -86.9348) centre (14.092, -86.884) ccw
  line L1941 (15.108, -86.884) -> (15.108, -88.916)
  arc A4230 (15.0572, -88.916) -> (15.1588, -88.916) centre (15.108, -88.916) ccw
  arc A4231 (15.1588, -86.884) -> (15.0572, -86.884) centre (15.108, -86.884) ccw
  line L1942 (15.108, -88.916) -> (14.092, -88.916)
  arc A4232 (14.092, -88.8652) -> (14.092, -88.9668) centre (14.092, -88.916) ccw
  arc A4233 (15.108, -88.9668) -> (15.108, -88.8652) centre (15.108, -88.916) ccw
  line L1943 (16.284, -79.292) -> (18.316, -79.292)
  arc A4234 (18.316, -79.3428) -> (18.316, -79.2412) centre (18.316, -79.292) ccw
  arc A4235 (16.284, -79.2412) -> (16.284, -79.3428) centre (16.284, -79.292) ccw
  line L1944 (18.316, -79.292) -> (18.316, -80.308)
  arc A4236 (18.2652, -80.308) -> (18.3668, -80.308) centre (18.316, -80.308) ccw
  arc A4237 (18.3668, -79.292) -> (18.2652, -79.292) centre (18.316, -79.292) ccw
  line L1945 (18.316, -80.308) -> (16.284, -80.308)
  arc A4238 (16.284, -80.2572) -> (16.284, -80.3588) centre (16.284, -80.308) ccw
  arc A4239 (18.316, -80.3588) -> (18.316, -80.2572) centre (18.316, -80.308) ccw
  line L1946 (16.284, -80.308) -> (16.284, -79.292)
  arc A4240 (16.3348, -79.292) -> (16.2332, -79.292) centre (16.284, -79.292) ccw
  arc A4241 (16.2332, -80.308) -> (16.3348, -80.308) centre (16.284, -80.308) ccw
  line L1947 (9.108, -87.684) -> (9.108, -89.716)
  arc A4242 (9.0572, -89.716) -> (9.1588, -89.716) centre (9.108, -89.716) ccw
  arc A4243 (9.1588, -87.684) -> (9.0572, -87.684) centre (9.108, -87.684) ccw
  line L1948 (9.108, -89.716) -> (8.092, -89.716)
  arc A4244 (8.092, -89.6652) -> (8.092, -89.7668) centre (8.092, -89.716) ccw
  arc A4245 (9.108, -89.7668) -> (9.108, -89.6652) centre (9.108, -89.716) ccw
  line L1949 (8.092, -89.716) -> (8.092, -87.684)
  arc A4246 (8.1428, -87.684) -> (8.0412, -87.684) centre (8.092, -87.684) ccw
  arc A4247 (8.0412, -89.716) -> (8.1428, -89.716) centre (8.092, -89.716) ccw
  line L1950 (8.092, -87.684) -> (9.108, -87.684)
  arc A4248 (9.108, -87.7348) -> (9.108, -87.6332) centre (9.108, -87.684) ccw
  arc A4249 (8.092, -87.6332) -> (8.092, -87.7348) centre (8.092, -87.684) ccw
  line L1951 (8.108, -87.684) -> (8.108, -89.716)
  arc A4250 (8.0572, -89.716) -> (8.1588, -89.716) centre (8.108, -89.716) ccw
  arc A4251 (8.1588, -87.684) -> (8.0572, -87.684) centre (8.108, -87.684) ccw
  line L1952 (8.108, -89.716) -> (7.092, -89.716)
  arc A4252 (7.092, -89.6652) -> (7.092, -89.7668) centre (7.092, -89.716) ccw
  arc A4253 (8.108, -89.7668) -> (8.108, -89.6652) centre (8.108, -89.716) ccw
  line L1953 (7.092, -89.716) -> (7.092, -87.684)
  arc A4254 (7.1428, -87.684) -> (7.0412, -87.684) centre (7.092, -87.684) ccw
  arc A4255 (7.0412, -89.716) -> (7.1428, -89.716) centre (7.092, -89.716) ccw
  line L1954 (7.092, -87.684) -> (8.108, -87.684)
  arc A4256 (8.108, -87.7348) -> (8.108, -87.6332) centre (8.108, -87.684) ccw
  arc A4257 (7.092, -87.6332) -> (7.092, -87.7348) centre (7.092, -87.684) ccw
  line L1955 (9.584, -80.392) -> (11.616, -80.392)
  arc A4258 (11.616, -80.4428) -> (11.616, -80.3412) centre (11.616, -80.392) ccw
  arc A4259 (9.584, -80.3412) -> (9.584, -80.4428) centre (9.584, -80.392) ccw
  line L1956 (11.616, -80.392) -> (11.616, -81.408)
  arc A4260 (11.5652, -81.408) -> (11.6668, -81.408) centre (11.616, -81.408) ccw
  arc A4261 (11.6668, -80.392) -> (11.5652, -80.392) centre (11.616, -80.392) ccw
  line L1957 (11.616, -81.408) -> (9.584, -81.408)
  arc A4262 (9.584, -81.3572) -> (9.584, -81.4588) centre (9.584, -81.408) ccw
  arc A4263 (11.616, -81.4588) -> (11.616, -81.3572) centre (11.616, -81.408) ccw
  line L1958 (9.584, -81.408) -> (9.584, -80.392)
  arc A4264 (9.6348, -80.392) -> (9.5332, -80.392) centre (9.584, -80.392) ccw
  arc A4265 (9.5332, -81.408) -> (9.6348, -81.408) centre (9.584, -81.408) ccw
  line L1959 (16.284, -81.192) -> (18.316, -81.192)
  arc A4266 (18.316, -81.2428) -> (18.316, -81.1412) centre (18.316, -81.192) ccw
  arc A4267 (16.284, -81.1412) -> (16.284, -81.2428) centre (16.284, -81.192) ccw
  line L1960 (18.316, -81.192) -> (18.316, -82.208)
  arc A4268 (18.2652, -82.208) -> (18.3668, -82.208) centre (18.316, -82.208) ccw
  arc A4269 (18.3668, -81.192) -> (18.2652, -81.192) centre (18.316, -81.192) ccw
  line L1961 (18.316, -82.208) -> (16.284, -82.208)
  arc A4270 (16.284, -82.1572) -> (16.284, -82.2588) centre (16.284, -82.208) ccw
  arc A4271 (18.316, -82.2588) -> (18.316, -82.1572) centre (18.316, -82.208) ccw
  line L1962 (16.284, -82.208) -> (16.284, -81.192)
  arc A4272 (16.3348, -81.192) -> (16.2332, -81.192) centre (16.284, -81.192) ccw
  arc A4273 (16.2332, -82.208) -> (16.3348, -82.208) centre (16.284, -82.208) ccw
  line L1963 (8.008, 12.216) -> (8.008, 10.184)
  arc A4274 (7.9572, 10.184) -> (8.0588, 10.184) centre (8.008, 10.184) ccw
  arc A4275 (8.0588, 12.216) -> (7.9572, 12.216) centre (8.008, 12.216) ccw
  line L1964 (8.008, 10.184) -> (6.992, 10.184)
  arc A4276 (6.992, 10.2348) -> (6.992, 10.1332) centre (6.992, 10.184) ccw
  arc A4277 (8.008, 10.1332) -> (8.008, 10.2348) centre (8.008, 10.184) ccw
  line L1965 (6.992, 10.184) -> (6.992, 12.216)
  arc A4278 (7.0428, 12.216) -> (6.9412, 12.216) centre (6.992, 12.216) ccw
  arc A4279 (6.9412, 10.184) -> (7.0428, 10.184) centre (6.992, 10.184) ccw
  line L1966 (6.992, 12.216) -> (8.008, 12.216)
  arc A4280 (8.008, 12.1652) -> (8.008, 12.2668) centre (8.008, 12.216) ccw
  arc A4281 (6.992, 12.2668) -> (6.992, 12.1652) centre (6.992, 12.216) ccw
  line L1967 (21.616, -90.508) -> (19.584, -90.508)
  arc A4282 (19.584, -90.4572) -> (19.584, -90.5588) centre (19.584, -90.508) ccw
  arc A4283 (21.616, -90.5588) -> (21.616, -90.4572) centre (21.616, -90.508) ccw
  line L1968 (19.584, -90.508) -> (19.584, -89.492)
  arc A4284 (19.6348, -89.492) -> (19.5332, -89.492) centre (19.584, -89.492) ccw
  arc A4285 (19.5332, -90.508) -> (19.6348, -90.508) centre (19.584, -90.508) ccw
  line L1969 (19.584, -89.492) -> (21.616, -89.492)
  arc A4286 (21.616, -89.5428) -> (21.616, -89.4412) centre (21.616, -89.492) ccw
  arc A4287 (19.584, -89.4412) -> (19.584, -89.5428) centre (19.584, -89.492) ccw
  line L1970 (21.616, -89.492) -> (21.616, -90.508)
  arc A4288 (21.5652, -90.508) -> (21.6668, -90.508) centre (21.616, -90.508) ccw
  arc A4289 (21.6668, -89.492) -> (21.5652, -89.492) centre (21.616, -89.492) ccw
  line L1971 (17.392, -118.716) -> (17.392, -116.684)
  arc A4290 (17.4428, -116.684) -> (17.3412, -116.684) centre (17.392, -116.684) ccw
  arc A4291 (17.3412, -118.716) -> (17.4428, -118.716) centre (17.392, -118.716) ccw
  line L1972 (17.392, -116.684) -> (18.408, -116.684)
  arc A4292 (18.408, -116.7348) -> (18.408, -116.6332) centre (18.408, -116.684) ccw
  arc A4293 (17.392, -116.6332) -> (17.392, -116.7348) centre (17.392, -116.684) ccw
  line L1973 (18.408, -116.684) -> (18.408, -118.716)
  arc A4294 (18.3572, -118.716) -> (18.4588, -118.716) centre (18.408, -118.716) ccw
  arc A4295 (18.4588, -116.684) -> (18.3572, -116.684) centre (18.408, -116.684) ccw
  line L1974 (18.408, -118.716) -> (17.392, -118.716)
  arc A4296 (17.392, -118.6652) -> (17.392, -118.7668) centre (17.392, -118.716) ccw
  arc A4297 (18.408, -118.7668) -> (18.408, -118.6652) centre (18.408, -118.716) ccw
  line L1975 (16.392, -118.716) -> (16.392, -116.684)
  arc A4298 (16.4428, -116.684) -> (16.3412, -116.684) centre (16.392, -116.684) ccw
  arc A4299 (16.3412, -118.716) -> (16.4428, -118.716) centre (16.392, -118.716) ccw
  line L1976 (16.392, -116.684) -> (17.408, -116.684)
  arc A4300 (17.408, -116.7348) -> (17.408, -116.6332) centre (17.408, -116.684) ccw
  arc A4301 (16.392, -116.6332) -> (16.392, -116.7348) centre (16.392, -116.684) ccw
  line L1977 (17.408, -116.684) -> (17.408, -118.716)
  arc A4302 (17.3572, -118.716) -> (17.4588, -118.716) centre (17.408, -118.716) ccw
  arc A4303 (17.4588, -116.684) -> (17.3572, -116.684) centre (17.408, -116.684) ccw
  line L1978 (17.408, -118.716) -> (16.392, -118.716)
  arc A4304 (16.392, -118.6652) -> (16.392, -118.7668) centre (16.392, -118.716) ccw
  arc A4305 (17.408, -118.7668) -> (17.408, -118.6652) centre (17.408, -118.716) ccw
  line L1979 (15.216, -107.908) -> (13.184, -107.908)
  arc A4306 (13.184, -107.8572) -> (13.184, -107.9588) centre (13.184, -107.908) ccw
  arc A4307 (15.216, -107.9588) -> (15.216, -107.8572) centre (15.216, -107.908) ccw
  line L1980 (13.184, -107.908) -> (13.184, -106.892)
  arc A4308 (13.2348, -106.892) -> (13.1332, -106.892) centre (13.184, -106.892) ccw
  arc A4309 (13.1332, -107.908) -> (13.2348, -107.908) centre (13.184, -107.908) ccw
  line L1981 (13.184, -106.892) -> (15.216, -106.892)
  arc A4310 (15.216, -106.9428) -> (15.216, -106.8412) centre (15.216, -106.892) ccw
  arc A4311 (13.184, -106.8412) -> (13.184, -106.9428) centre (13.184, -106.892) ccw
  line L1982 (15.216, -106.892) -> (15.216, -107.908)
  arc A4312 (15.1652, -107.908) -> (15.2668, -107.908) centre (15.216, -107.908) ccw
  arc A4313 (15.2668, -106.892) -> (15.1652, -106.892) centre (15.216, -106.892) ccw
  line L1983 (13.184, -107.892) -> (15.216, -107.892)
  arc A4314 (15.216, -107.9428) -> (15.216, -107.8412) centre (15.216, -107.892) ccw
  arc A4315 (13.184, -107.8412) -> (13.184, -107.9428) centre (13.184, -107.892) ccw
  line L1984 (15.216, -107.892) -> (15.216, -108.908)
  arc A4316 (15.1652, -108.908) -> (15.2668, -108.908) centre (15.216, -108.908) ccw
  arc A4317 (15.2668, -107.892) -> (15.1652, -107.892) centre (15.216, -107.892) ccw
  line L1985 (15.216, -108.908) -> (13.184, -108.908)
  arc A4318 (13.184, -108.8572) -> (13.184, -108.9588) centre (13.184, -108.908) ccw
  arc A4319 (15.216, -108.9588) -> (15.216, -108.8572) centre (15.216, -108.908) ccw
  line L1986 (13.184, -108.908) -> (13.184, -107.892)
  arc A4320 (13.2348, -107.892) -> (13.1332, -107.892) centre (13.184, -107.892) ccw
  arc A4321 (13.1332, -108.908) -> (13.2348, -108.908) centre (13.184, -108.908) ccw
  line L1987 (12.997, -109.035) -> (10.203, -109.035)
  arc A4322 (10.203, -108.9842) -> (10.203, -109.0858) centre (10.203, -109.035) ccw
  arc A4323 (12.997, -109.0858) -> (12.997, -108.9842) centre (12.997, -109.035) ccw
  line L1988 (10.203, -109.035) -> (10.203, -107.765)
  arc A4324 (10.2538, -107.765) -> (10.1522, -107.765) centre (10.203, -107.765) ccw
  arc A4325 (10.1522, -109.035) -> (10.2538, -109.035) centre (10.203, -109.035) ccw
  line L1989 (10.203, -107.765) -> (12.997, -107.765)
  arc A4326 (12.997, -107.8158) -> (12.997, -107.7142) centre (12.997, -107.765) ccw
  arc A4327 (10.203, -107.7142) -> (10.203, -107.8158) centre (10.203, -107.765) ccw
  line L1990 (12.997, -107.765) -> (12.997, -109.035)
  arc A4328 (12.9462, -109.035) -> (13.0478, -109.035) centre (12.997, -109.035) ccw
  arc A4329 (13.0478, -107.765) -> (12.9462, -107.765) centre (12.997, -107.765) ccw
  line L1991 (19.892, -118.716) -> (19.892, -116.684)
  arc A4330 (19.9428, -116.684) -> (19.8412, -116.684) centre (19.892, -116.684) ccw
  arc A4331 (19.8412, -118.716) -> (19.9428, -118.716) centre (19.892, -118.716) ccw
  line L1992 (19.892, -116.684) -> (20.908, -116.684)
  arc A4332 (20.908, -116.7348) -> (20.908, -116.6332) centre (20.908, -116.684) ccw
  arc A4333 (19.892, -116.6332) -> (19.892, -116.7348) centre (19.892, -116.684) ccw
  line L1993 (20.908, -116.684) -> (20.908, -118.716)
  arc A4334 (20.8572, -118.716) -> (20.9588, -118.716) centre (20.908, -118.716) ccw
  arc A4335 (20.9588, -116.684) -> (20.8572, -116.684) centre (20.908, -116.684) ccw
  line L1994 (20.908, -118.716) -> (19.892, -118.716)
  arc A4336 (19.892, -118.6652) -> (19.892, -118.7668) centre (19.892, -118.716) ccw
  arc A4337 (20.908, -118.7668) -> (20.908, -118.6652) centre (20.908, -118.716) ccw
  line L1995 (5.065, -108.897) -> (5.065, -106.103)
  arc A4338 (5.1158, -106.103) -> (5.0142, -106.103) centre (5.065, -106.103) ccw
  arc A4339 (5.0142, -108.897) -> (5.1158, -108.897) centre (5.065, -108.897) ccw
  line L1996 (5.065, -106.103) -> (6.335, -106.103)
  arc A4340 (6.335, -106.1538) -> (6.335, -106.0522) centre (6.335, -106.103) ccw
  arc A4341 (5.065, -106.0522) -> (5.065, -106.1538) centre (5.065, -106.103) ccw
  line L1997 (6.335, -106.103) -> (6.335, -108.897)
  arc A4342 (6.2842, -108.897) -> (6.3858, -108.897) centre (6.335, -108.897) ccw
  arc A4343 (6.3858, -106.103) -> (6.2842, -106.103) centre (6.335, -106.103) ccw
  line L1998 (6.335, -108.897) -> (5.065, -108.897)
  arc A4344 (5.065, -108.8462) -> (5.065, -108.9478) centre (5.065, -108.897) ccw
  arc A4345 (6.335, -108.9478) -> (6.335, -108.8462) centre (6.335, -108.897) ccw
  line L1999 (3.665, -108.897) -> (3.665, -106.103)
  arc A4346 (3.7158, -106.103) -> (3.6142, -106.103) centre (3.665, -106.103) ccw
  arc A4347 (3.6142, -108.897) -> (3.7158, -108.897) centre (3.665, -108.897) ccw
  line L2000 (3.665, -106.103) -> (4.935, -106.103)
  arc A4348 (4.935, -106.1538) -> (4.935, -106.0522) centre (4.935, -106.103) ccw
  arc A4349 (3.665, -106.0522) -> (3.665, -106.1538) centre (3.665, -106.103) ccw
  line L2001 (4.935, -106.103) -> (4.935, -108.897)
  arc A4350 (4.8842, -108.897) -> (4.9858, -108.897) centre (4.935, -108.897) ccw
  arc A4351 (4.9858, -106.103) -> (4.8842, -106.103) centre (4.935, -106.103) ccw
  line L2002 (4.935, -108.897) -> (3.665, -108.897)
  arc A4352 (3.665, -108.8462) -> (3.665, -108.9478) centre (3.665, -108.897) ccw
  arc A4353 (4.935, -108.9478) -> (4.935, -108.8462) centre (4.935, -108.897) ccw
  line L2003 (7.392, -108.116) -> (7.392, -106.084)
  arc A4354 (7.4428, -106.084) -> (7.3412, -106.084) centre (7.392, -106.084) ccw
  arc A4355 (7.3412, -108.116) -> (7.4428, -108.116) centre (7.392, -108.116) ccw
  line L2004 (7.392, -106.084) -> (8.408, -106.084)
  arc A4356 (8.408, -106.1348) -> (8.408, -106.0332) centre (8.408, -106.084) ccw
  arc A4357 (7.392, -106.0332) -> (7.392, -106.1348) centre (7.392, -106.084) ccw
  line L2005 (8.408, -106.084) -> (8.408, -108.116)
  arc A4358 (8.3572, -108.116) -> (8.4588, -108.116) centre (8.408, -108.116) ccw
  arc A4359 (8.4588, -106.084) -> (8.3572, -106.084) centre (8.408, -106.084) ccw
  line L2006 (8.408, -108.116) -> (7.392, -108.116)
  arc A4360 (7.392, -108.0652) -> (7.392, -108.1668) centre (7.392, -108.116) ccw
  arc A4361 (8.408, -108.1668) -> (8.408, -108.0652) centre (8.408, -108.116) ccw
  line L2007 (-10.816, -103.592) -> (-8.784, -103.592)
  arc A4362 (-8.784, -103.6428) -> (-8.784, -103.5412) centre (-8.784, -103.592) ccw
  arc A4363 (-10.816, -103.5412) -> (-10.816, -103.6428) centre (-10.816, -103.592) ccw
  line L2008 (-8.784, -103.592) -> (-8.784, -104.608)
  arc A4364 (-8.8348, -104.608) -> (-8.7332, -104.608) centre (-8.784, -104.608) ccw
  arc A4365 (-8.7332, -103.592) -> (-8.8348, -103.592) centre (-8.784, -103.592) ccw
  line L2009 (-8.784, -104.608) -> (-10.816, -104.608)